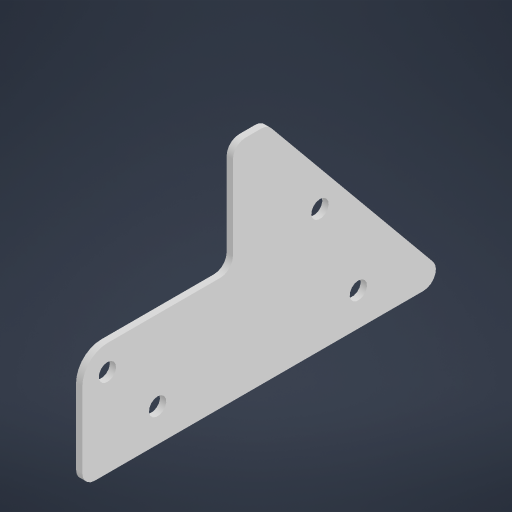
# Autodesk Inventor part: sledsv3
Saved by Autodesk Inventor 2024 (Build 280153000, 153)
## iProperties
Created: 2023-12-14
Part Number: sledsv3
Material: Generic
Document SubType Name: Sheet Metal
Designer: reima
Density: 1 g/cm^3
Sheet Metal Rule: Default
Appearance: Default
Author: reima
Autodesk Inventor part; units mm, degrees
ref_plane "YZ Plane" through (0, 0, 0) normal (1, 0, 0) x (0, 1, 0)
ref_plane "XZ Plane" through (0, 0, 0) normal (0, 1, 0) x (-1, 0, 0)
ref_plane "XY Plane" through (0, 0, 0) normal (0, 0, 1) x (1, 0, 0)
sketch "Sketch1" plane through (0, 0, 0) normal (1, 0, 0) x (0, 1, 0)
  line L0 (3.1935, -18.6702) -> (3.1935, -95.8243)
  arc A0 (3.1935, -95.8243) -> (7.9971, -98.5498) centre (6.3685, -95.8243) ccw
  arc A1 (7.9971, -98.5498) -> (58.1414, -63.3045) centre (-204.4103, 256.9406) ccw
  arc A2 (58.1414, -63.3045) -> (59.3034, -60.8492) centre (56.1284, -60.8492) ccw
  line L1 (59.3034, -60.8492) -> (59.3034, -56.7702)
  arc A3 (59.3034, -56.7702) -> (56.1284, -53.5952) centre (56.1284, -56.7702) ccw
  line L2 (56.1284, -53.5952) -> (34.9435, -53.5952)
  arc A4 (31.7685, -50.4202) -> (34.9435, -53.5952) centre (34.9435, -50.4202) ccw
  line L3 (31.7685, -50.4202) -> (31.7685, -21.8452)
  arc A5 (31.7685, -21.8452) -> (25.4185, -15.4952) centre (25.4185, -21.8452) ccw
  line L4 (25.4185, -15.4952) -> (6.3685, -15.4952)
  arc A6 (6.3685, -15.4952) -> (3.1935, -18.6702) centre (6.3685, -18.6702) ccw
  circle A7 centre (11.5501, -34.5452) radius 2.1844
  circle A8 centre (11.5501, -85.3452) radius 2.1844
  circle A9 centre (34.2518, -75.6387) radius 2.1844
  circle A10 centre (25.4185, -21.8452) radius 2.1844
  point P0 (0, 0)
  point P1 (25.4185, -15.4952)
  point P2 (3.1935, -18.6702)
  point P3 (7.9971, -98.5498)
  point P4 (58.1414, -63.3045)
  point P5 (34.9435, -53.5952)
sketch "Sketch2" plane through (1.5875, 0, 0) normal (1, 0, 0) x (0, 0, -1)
  line L0 (18.6702, 3.1935) -> (95.8243, 3.1935)
  line L1 (95.8243, 3.1935) -> (101.7995, 3.1935)
  arc A0 (63.3045, 58.1414) -> (60.8492, 59.3034) centre (60.8492, 56.1284) ccw
  line L2 (104.251, 8.3861) -> (63.3045, 58.1414)
  arc A1 (101.7995, 3.1935) -> (104.251, 8.3861) centre (101.7995, 6.3685) ccw
  arc A2 (98.5498, 7.9971) -> (63.3045, 58.1414) centre (-256.9406, -204.4103) ccw
  arc A3 (95.8243, 3.1935) -> (98.5498, 7.9971) centre (95.8243, 6.3685) ccw
  point P0 (0, 0)
  point P1 (108.5243, 3.1935)
  dimension "d1" = 12.7
  dimension "d2" = 3.175
  measures "d1" distance of L0.end point (108.524, 3.194)
  measures "d2" radius of A1
extrude "Plate1" add sketch "Sketch1" along normal blind 1.5875
sheet face with bend "Face2" sketch "Sketch2" thickness 1.5875 toward (-1, 0, 0) bend radius 1.5875
bend "Bend1"
equation "\"d0\" = Thickness"
equation "\"d3\" = BendRadius"
equation "\"d4\" = BendReliefWidth"
equation "\"d6\" = MinimumRemnant"
equation "\"d5\" = BendReliefDepth"
equation "\"d7\" = TransitionRadius"
equation "\"BendRadius\" = Thickness"
equation "\"BendReliefWidth\" = Thickness"
equation "\"BendReliefDepth\" = 0.5 * Thickness"
equation "\"CornerReliefSize\" = 4 * Thickness"
equation "\"MinimumRemnant\" = 2 * Thickness"
equation "\"TransitionRadius\" = BendRadius"
equation "\"JacobiRadiusSize\" = BendRadius"
equation "\"GapSize\" = Thickness"
equation "\"Thickness\" = 1.5875"
body "Solid1"
